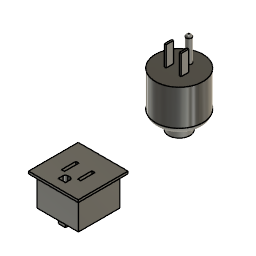
nema (Autodesk Fusion 360 design; units mm, degrees)
part number: 2026-03-30-18-51-31-380
Autodesk Fusion 360 part; units mm, degrees
sketch "Boceto1" plane through (0, 0, 0) normal (0, 0, 1) x (1, 0, 0)
  circle A0 centre (75, 55) radius 20
  dimension "d1" = 40
  measures "d1" diameter of A0
extrude "Extruir1" add sketch "Boceto1" along normal blind 35 makes body 1
fillet "Empalme1" radius 5 1 faces at (63.8127, 57.6911, 0) on bodies 1
sketch "Boceto2" plane through (0, 0, 35) normal (0, 0, 1) x (-1, 0, 0)
  circle A0 centre (-75, -55) radius 20
  circle A1 centre (-75, -63.1) radius 2.4
  line L0 (-75, -75) -> (-75, -63.1)
  line L1 (-80.7445, -55.7276) -> (-82.2445, -55.7276)
  line L2 (-82.2445, -55.7276) -> (-82.2445, -49.4276)
  line L3 (-82.2445, -49.4276) -> (-80.7445, -49.4276)
  line L4 (-80.7445, -49.4276) -> (-80.7445, -55.7276)
  line L5 (-80.7445, -55.7276) -> (-82.2445, -49.4276) construction
  line L6 (-82.2445, -55.7276) -> (-80.7445, -49.4276) construction
  line L7 (-81.4945, -52.5776) -> (-68.7945, -52.5776)
  line L8 (-68.0445, -55.7276) -> (-69.5445, -55.7276)
  line L9 (-69.5445, -55.7276) -> (-69.5445, -49.4276)
  line L10 (-69.5445, -49.4276) -> (-68.0445, -49.4276)
  line L11 (-68.0445, -49.4276) -> (-68.0445, -55.7276)
  line L12 (-68.0445, -55.7276) -> (-69.5445, -49.4276) construction
  line L13 (-69.5445, -55.7276) -> (-68.0445, -49.4276) construction
  line L14 (-75, -35) -> (-75, -56.7166)
  point P0 (-81.4945, -52.5776)
  point P1 (-68.7945, -52.5776)
  dimension "d6" = 4.8
  dimension "d7" = 11.9
  dimension "d8" = 1.5
  dimension "d9" = 6.3
  dimension "d10" = 12.7
  dimension "d11" = 1.5
  dimension "d12" = 6.3
  constraint coincident A0 L0.start
  constraint vertical L0
  constraint coincident A1.centre L0.end
  constraint horizontal L1
  constraint perpendicular L1 L2
  constraint parallel L1 L3
  constraint parallel L2 L4
  constraint coincident L5 P0
  constraint coincident L6 P0
  constraint coincident P0 L7.start
  constraint perpendicular L4 L7
  constraint horizontal L8
  constraint perpendicular L8 L9
  constraint parallel L8 L10
  constraint parallel L9 L11
  constraint coincident L12 P1
  constraint coincident L13 P1
  constraint coincident P1 L7.end
  constraint coincident A0 L14.start
  constraint vertical L14
  measures "d6" diameter of A1
  measures "d7" distance of L0.start A1.centre
  measures "d8" distance of L2.end L3.end
  measures "d9" distance of L1.end L2.end
  measures "d10" distance of P0 P1
  measures "d11" distance of L9.end L10.end
  measures "d12" distance of L8.end L9.end
extrude "Extruir2" add sketch "Boceto2" along normal blind 17 contours L1 L2 L3 L4 | L8 L9 L10 L11 bodies 1
extrude "Extruir3" add sketch "Boceto2" along normal blind 21 contours A1 bodies 1
fillet "Empalme2" radius 2 1 faces at (74.5012, 62.0029, 56) on bodies 1
sketch "Boceto3" plane through (0, 0, 0) normal (0, 0, -1) x (1, 0, 0)
  circle A0 centre (75, -55) radius 15
  circle A1 centre (75, -55) radius 9
  dimension "d19" = 18
  constraint concentric A0 A1
  measures "d19" diameter of A1
extrude "Extruir4" add sketch "Boceto3" along normal blind 10 contours A1 bodies 1
sketch "Boceto10" plane through (0, 0, 0) normal (0, 0, 1) x (1, 0, 0)
  line L0 (95.7817, -50.9127) -> (53.7817, -50.9127)
  line L1 (53.7817, -50.9127) -> (53.7817, -8.9127)
  line L2 (53.7817, -8.9127) -> (95.7817, -8.9127)
  line L3 (95.7817, -8.9127) -> (95.7817, -50.9127)
  line L4 (95.7817, -50.9127) -> (53.7817, -8.9127) construction
  line L5 (53.7817, -50.9127) -> (95.7817, -8.9127) construction
  line L6 (74.7817, -8.9127) -> (74.7817, -29.9127)
  line L7 (95.7817, -29.9127) -> (74.7817, -29.9127)
  line L8 (85.2817, -29.9127) -> (85.2817, -8.9127)
  line L9 (85.2817, -29.9127) -> (65, -29.9127)
  line L10 (69.201, -35.9127) -> (66.701, -35.9127)
  line L11 (66.701, -35.9127) -> (66.701, -23.9127)
  line L12 (66.701, -23.9127) -> (69.201, -23.9127)
  line L13 (69.201, -23.9127) -> (69.201, -35.9127)
  line L14 (69.201, -35.9127) -> (66.701, -23.9127) construction
  line L15 (66.701, -35.9127) -> (69.201, -23.9127) construction
  line L16 (80.3485, -23.9127) -> (82.8485, -23.9127)
  line L17 (82.8485, -23.9127) -> (82.8485, -35.9127)
  line L18 (82.8485, -35.9127) -> (80.3485, -35.9127)
  line L19 (80.3485, -35.9127) -> (80.3485, -23.9127)
  line L20 (80.3485, -23.9127) -> (82.8485, -35.9127) construction
  line L21 (82.8485, -23.9127) -> (80.3485, -35.9127) construction
  line L22 (77.7817, -43.6849) -> (71.7817, -43.6849)
  line L23 (71.7817, -43.6849) -> (71.7817, -39.6849)
  line L24 (73.7817, -37.6849) -> (75.7817, -37.6849)
  line L25 (77.7817, -39.6849) -> (77.7817, -43.6849)
  line L26 (77.7817, -43.6849) -> (71.7817, -37.6849) construction
  line L27 (71.7817, -43.6849) -> (77.7817, -37.6849) construction
  arc A0 (73.7817, -37.6849) -> (71.7817, -39.6849) centre (73.7817, -39.6849) ccw
  arc A1 (77.7817, -39.6849) -> (75.7817, -37.6849) centre (75.7817, -39.6849) ccw
  line L28 (57.3512, -47.3433) -> (92.3512, -47.3433)
  line L29 (92.3512, -47.3433) -> (92.3512, -12.3433)
  line L30 (92.3512, -12.3433) -> (57.3512, -12.3433)
  line L31 (57.3512, -12.3433) -> (57.3512, -47.3433)
  point P0 (74.7817, -29.9127)
  point P1 (67.951, -29.9127)
  point P2 (81.5985, -29.9127)
  point P3 (74.7817, -40.6849)
  dimension "d56" = 42
  dimension "d57" = 42
  dimension "d58" = 2.5
  dimension "d59" = 12
  dimension "d60" = 2.5
  dimension "d61" = 12
  dimension "d62" = 6
  dimension "d63" = 6
  dimension "d64" = 2
  dimension "d65" = 2
  dimension "d68" = 35
  dimension "d69" = 35
  constraint horizontal L0
  constraint perpendicular L0 L1
  constraint parallel L0 L2
  constraint parallel L1 L3
  constraint coincident L4 P0
  constraint coincident L5 P0
  constraint midpoint L2 L6.start
  constraint coincident P0 L6.end
  constraint midpoint L3 L7.start
  constraint midpoint L7 L8.start
  constraint coincident L2 L8.end
  constraint perpendicular L2 L8
  constraint perpendicular L6 L9
  constraint horizontal L10
  constraint perpendicular L10 L11
  constraint parallel L10 L12
  constraint parallel L11 L13
  constraint coincident L14 P1
  constraint coincident L15 P1
  constraint coincident L9 P1
  constraint horizontal L16
  constraint perpendicular L16 L17
  constraint parallel L16 L18
  constraint parallel L17 L19
  constraint coincident L20 P2
  constraint coincident L21 P2
  constraint coincident L7 P2
  constraint horizontal L22
  constraint perpendicular L22 L23
  constraint parallel L22 L24
  constraint parallel L23 L25
  constraint coincident L26 P3
  constraint coincident L27 P3
  constraint coincident L26.end L23
  constraint coincident L26.end L24
  constraint tangent L23 A0
  constraint tangent L24 A0
  constraint coincident L27.end L24
  constraint coincident L27.end L25
  constraint tangent L24 A1
  constraint tangent L25 A1
  constraint horizontal L28
  constraint vertical L29
  constraint horizontal L30
  constraint vertical L31
  constraint coincident L5 L28.start
  measures "d56" distance of L1.end L2.end
  measures "d57" distance of L0.end L1.end
  measures "d58" distance of L11.end L12.end
  measures "d59" distance of L10.end L11.end
  measures "d60" distance of L17.end L18.end
  measures "d61" distance of L16.end L17.end
  measures "d62" distance of L26.end L27.end
  measures "d63" distance of L22.end L26.end
  measures "d64" radius of A0
  measures "d65" radius of A1
  measures "d68" distance of L28.start L28.end
  measures "d69" distance of L28.start L30.end
extrude "Extruir11" add sketch "Boceto10" along normal blind 2 separate body contours L0 L1 L2 L3 L6 L7 L28 L29 L30 L31 | L2 L3 L7 L8 L29 L30 | L6 L7 L9 L17 L18 L19 L28 L29 L30 L31 | L7 L8 L29 L30 | L2 L6 L8 L30 | L6 L7 L8 L9 L16 L17 L19 L30 makes body 2
extrude "Extruir12" add sketch "Boceto10" against normal blind 25 separate body contours L6 L7 L9 L17 L18 L19 L28 L29 L30 L31 | L7 L8 L29 L30 | L6 L7 L8 L9 L16 L17 L19 L30 makes body 3
extrude "Extruir13" add sketch "Boceto10" against normal blind 31 contours L7 L9 L17 L18 L19 | L7 L9 L16 L17 L19 | L9 L10 L11 L13 | L9 L11 L12 L13 | L22 L23 L24 L25 A0 A1 bodies 2 3
extrude "Extruir14" cut 3 faces at (68.3677, -27.9127, 0) (81.1819, -27.9127, 0) (75.7817, -42.3516, 0) along direction (0, 0, -1) blind 19 on bodies 2 bodies 2
